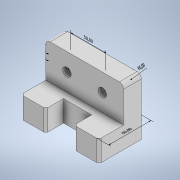
# Autodesk Inventor part: Część2
Saved by Autodesk Inventor 2021 (Build 250183000, 183)
## iProperties
Created: 2023-09-21
Part Number: Część2
Material: Ogólny
Document SubType Name: Modeling
Designer: Jakub
Density: 1 g/cm^3
Appearance: Domyślna
Author: Jakub
Autodesk Inventor part; units mm, degrees
ref_plane "YZ Plane" through (0, 0, 0) normal (1, 0, 0) x (0, 1, 0)
ref_plane "XZ Plane" through (0, 0, 0) normal (0, 1, 0) x (-1, 0, 0)
ref_plane "XY Plane" through (0, 0, 0) normal (0, 0, 1) x (1, 0, 0)
sketch "Szkic1" plane through (0, 0, 0) normal (0, 1, 0) x (-1, 0, 0)
  line L0 (0, 0) -> (0, -60)
  line L1 (0, -60) -> (-110, -60)
  line L2 (-110, -60) -> (-110, 0)
  line L3 (-110, 0) -> (-75, 0)
  line L4 (-75, 0) -> (-75, -25)
  line L5 (-75, -25) -> (-35, -25)
  line L6 (-35, -25) -> (-35, 0)
  line L7 (-35, 0) -> (0, 0)
  dimension "d0" = 60
  dimension "d1" = 110
  dimension "d2" = 35
  dimension "d3" = 25
  dimension "d4" = 40
  constraints: 16 end point, 6 perpendicular, 2 vertical
  measures "d0" distance of L0.start L0.end
  measures "d1" distance of L0.end L1.end
  measures "d2" distance of L2.end L3.end
  measures "d3" distance of L3.end L4.end
  measures "d4" distance of L4.end L5.end
extrude "Wyciągnięcie proste1" add sketch "Szkic1" along normal blind 30
chamfer "Faza1" distance 3 angle 45 1 edges at (0, 15, 0)
chamfer "Faza2" distance 3 angle 45 1 edges at (110, 15, 0)
chamfer "Faza3" distance 3 angle 45 1 edges at (35, 15, 0)
chamfer "Faza4" distance 3 angle 45 1 edges at (75, 15, 0)
sketch "Szkic2" plane through (0, 30, 0) normal (0, 1, 0) x (1, 0, 0)
  line L0 (0, 60) -> (0, 3) projected
  line L1 (0, 60) -> (0, 35)
  line L2 (0, 35) -> (110, 35)
  line L3 (110, 3) -> (110, 60) projected
  line L4 (110, 60) -> (0, 60) projected
  line L5 (110, 60) -> (0, 60)
  point P0 (0, 0)
  dimension "d19" = 25
  constraints: 6 end point, 2 point on line, 1 collinear, 1 perpendicular
  measures "d19" distance of L0.start L1.end
extrude "Wyciągnięcie proste2" add sketch "Szkic2" along normal blind 50
fillet "Zaokrąglenie1" radius 6 1 edges at (0, 80, -47.5)
fillet "Zaokrąglenie2" radius 6 1 edges at (110, 80, -47.5)
sketch "Szkic3" plane through (0, 30, -35) normal (0, 0, 1) x (1, 0, 0)
  arc A0 (6, 50) -> (0, 44) centre (6, 44) ccw projected
  line L0 (6, 50) -> (6, 25)
  line L1 (0, -30) -> (0, 44) projected
  line L2 (0, 25) -> (110, 25)
  line L3 (110, 0) -> (110, 44) projected
  line L4 (0, 44) -> (30, 44)
  line L5 (30, 44) -> (30, 25)
  circle A1 centre (30, 25) radius 6
  dimension "d24" = 25
  dimension "d25" = 30
  dimension "d26" = 12
  constraints: 8 end point, 3 point on line, 2 perpendicular, 1 centre point, 1 coincident, 1 horizontal, 1 vertical
  measures "d24" distance of L0.start L0.end
  measures "d25" distance of L1.end L4.end
  measures "d26" diameter of A1
extrude "Wyciągnięcie proste3" cut sketch "Szkic3" against normal blind 5 contours A1 L5 L2 | L2 A1 | A1 L2 L5
sketch "Szkic4" plane through (0, 30, -35) normal (0, 0, 1) x (1, 0, 0)
  line L0 (0, 0) -> (0, 44) projected
  line L1 (0, 25) -> (110.0465, 25)
  line L2 (110.0465, 25) -> (110.0465, 50)
  line L3 (110.0465, 50) -> (30.0465, 50)
  line L4 (6, 50) -> (104, 50) projected
  line L5 (30.0465, 50) -> (30.0465, 0)
  line L6 (110, 0) -> (0, 0) projected
  line L7 (80, 50) -> (80, 0)
  circle A0 centre (80, 25) radius 6
  circle A1 centre (30.0465, 25) radius 3
  point P0 (0, -30)
  dimension "d29" = 80
  dimension "d30" = 12
  dimension "d31" = 6
  constraints: 10 end point, 4 point on line, 2 centre point, 2 midpoint, 2 perpendicular, 1 horizontal, 1 vertical
  measures "d29" distance of L2.end L3.end
  measures "d30" diameter of A0
  measures "d31" diameter of A1
extrude "Wyciągnięcie proste4" cut sketch "Szkic4" against normal blind 5 contours A0 L1 L7 | L7 L1 A0 | A0 L7 L1 | L7 A0 L1
sketch "Szkic5" plane through (0, 30, -35) normal (0, 0, 1) x (1, 0, 0)
  line L0 (110, 0) -> (110, 44) projected
  line L1 (110, 25) -> (0, 25)
  line L2 (0, 25) -> (0, 50)
  line L3 (0, 50) -> (30, 50)
  line L4 (6, 50) -> (104, 50) projected
  line L5 (30, 50) -> (30, 25)
  point P0 (0, -30)
  dimension "d34" = 30
  constraints: 8 end point, 3 point on line, 2 perpendicular, 1 horizontal
  measures "d34" distance of L2.end L3.end
hole "Otwór1" at (30, 55, -35) direction (0, 0, -1) diameter 6 depth 28.228 tip angle 118
sketch "Szkic6" plane through (110, 0, -60) normal (0, 0, -1) x (-1, 0, 0)
  point P0 (110, 0)
sketch "Szkic7" plane through (110, 0, -60) normal (0, 0, -1) x (-1, 0, 0)
  point P0 (110, 0)
sketch "Szkic8" plane through (110, 0, -60) normal (0, 0, -1) x (-1, 0, 0)
  line L0 (104, 80) -> (6, 80) projected
  line L1 (30, 80) -> (30, 6.837)
  circle A0 centre (30, 55) radius 6 projected
  line L2 (30, 6.837) -> (30, 55)
  line L3 (30, 55) -> (0, 55)
  line L4 (0, 30) -> (0, 74) projected
  line L5 (110, 30) -> (110, 74) projected
  line L6 (110, 55) -> (30, 55)
  point P0 (110, 0)
  constraints: 8 end point, 4 point on line, 2 collinear, 1 perpendicular, 1 vertical
hole "Otwór2" at (80, 55, -60) direction (0, 0, 1) diameter 6 depth 28.228 tip angle 118
